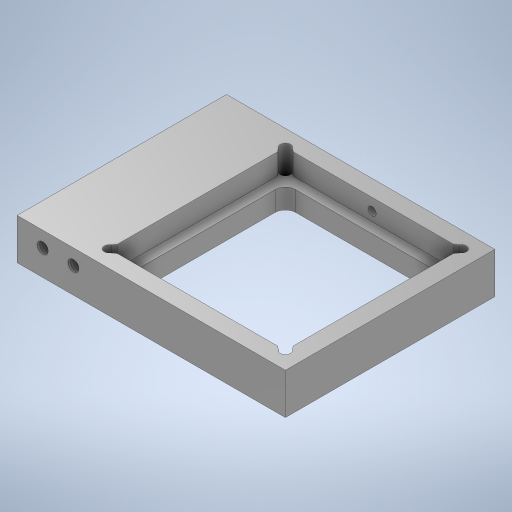
# Autodesk Inventor part: MirrorHolder
Saved by Autodesk Inventor 2023 (Build 270158000, 158)
## iProperties
Created: 2021-10-06
Part Number: MirrorHolder
Material: Aluminum 6061
Document SubType Name: Modeling
Designer: Timo
Density: 2.7 g/cm^3
Appearance: Anodized - Light Gray
Author: Timo
Autodesk Inventor part; units mm, degrees
ref_plane "YZ Plane" through (0, 0, 0) normal (1, 0, 0) x (0, 1, 0)
ref_plane "XZ Plane" through (0, 0, 0) normal (0, 1, 0) x (-1, 0, 0)
ref_plane "XY Plane" through (0, 0, 0) normal (0, 0, 1) x (1, 0, 0)
sketch "Sketch1" plane through (0, 0, 0) normal (0, 1, 0) x (-1, 0, 0)
  line L0 (12, 0) -> (-66.5, 0)
  line L1 (-66.5, 0) -> (-66.5, -61.3)
  line L2 (-66.5, -61.3) -> (12, -61.3)
  line L3 (12, -61.3) -> (12, 0)
  point P0 (0, 0)
  dimension "d0" = 12
  dimension "d1" = 66.5
  dimension "d2" = 61.3
  constraints: 8 end point, 2 parallel, 1 horizontal, 1 perpendicular, 1 point on line
  measures "d0" distance from line of L3 point (0, 0)
  measures "d1" distance from line of L1 point (0, 0)
  measures "d2" distance of L0.end L1.end
extrude "Extrusion1" add sketch "Sketch1" against normal blind 12
sketch "Sketch2" plane through (0, 0, 0) normal (0, 1, 0) x (1, 0, 0)
  line L0 (61.5, 56.5) -> (10, 56.5)
  line L1 (10, 56.5) -> (10, 5)
  line L2 (10, 5) -> (61.5, 5)
  line L3 (61.5, 5) -> (61.5, 56.5)
  line L4 (-12, 0) -> (66.5, 0) projected
  point P0 (0, 0)
  dimension "d5" = 10
  dimension "d6" = 51.5
  dimension "d7" = 5
  dimension "d8" = 51.5
  constraints: 8 end point, 2 parallel, 1 horizontal, 1 perpendicular
  measures "d5" distance from line of point (0, 0) L1
  measures "d6" distance of L2.end L0.start
  measures "d7" distance between parallel lines of L4 L2
  measures "d8" distance of L0.start L0.end
extrude "Extrusion2" cut sketch "Sketch2" against normal blind 6.2
sketch "Sketch3" plane through (0, 0, 0) normal (0, 1, 0) x (1, 0, 0)
  line L0 (61.5, 5) -> (10, 5) projected
  circle A0 centre (10, 5) radius 1.5
  circle A1 centre (61.5, 5) radius 1.5
  line L1 (10, 56.5) -> (61.5, 56.5) projected
  circle A2 centre (61.5, 56.5) radius 1.5
  circle A3 centre (10, 56.5) radius 1.5
  point P0 (0, 0)
  dimension "d11" = 3
  constraints: 4 centre point, 3 equal radius, 2 coincident
  measures "d11" diameter of A0
extrude "Extrusion3" cut sketch "Sketch3" against normal through all
chamfer "Chamfer1" distance 0.8 angle 45 8 edges at (10, -3.1, -6.5) (10, -3.1, -55) (11.5, -3.1, -56.5) (60, -3.1, -56.5) (61.5, -3.1, -55) (61.5, -3.1, -6.5) (60, -3.1, -5) (11.5, -3.1, -5)
sketch "Sketch4" plane through (0, -6.2, 0) normal (0, 1, 0) x (1, 0, 0)
  arc A0 (9.229, 55.2133) -> (11.2867, 57.271) centre (10, 56.5) ccw construction
  line L0 (10, 56.5) -> (61.5, 56.5) construction
  line L1 (61.5, 56.5) -> (61.5, 5) construction
  line L2 (61.5, 5) -> (10, 5) construction
  line L3 (10, 5) -> (10, 56.5) construction
  arc A1 (60.2133, 4.229) -> (62.271, 6.2867) centre (61.5, 5) ccw construction
  line L4 (58.5, 8) -> (58.5, 53.5) construction
  line L5 (58.5, 53.5) -> (13, 53.5) construction
  line L6 (13, 53.5) -> (13, 8) construction
  line L7 (13, 8) -> (58.5, 8) construction
  line L8 (13, 8) -> (58.5, 8)
  line L9 (58.5, 8) -> (58.5, 53.5)
  line L10 (58.5, 53.5) -> (13, 53.5)
  line L11 (13, 53.5) -> (13, 8)
  point P0 (0, 0)
  dimension "d19" = 3
  constraints: 24 end point, 6 parallel, 3 perpendicular, 2 horizontal, 1 coincident, 3 other
  measures "d19" distance between parallel lines of L1 L4
extrude "Extrusion4" cut sketch "Sketch4" against normal blind 6.2
fillet "Fillet1" radius 3 4 edges at (13, -9.1, -53.5) (58.5, -9.1, -8) (13, -9.1, -8) (58.5, -9.1, -53.5)
sketch "Sketch5" plane through (66.5, 0, -61.3) normal (0, 0, -1) x (-1, 0, 0)
  line L0 (0, 0) -> (78.5, 0) projected
  point P0 (66.5, 0)
  point P1 (31.1, -3.5)
  point P2 (56.5, -6.2)
  dimension "d24" = 25.4
  dimension "d25" = 3.5
  measures "d24" horizontal distance of point (56.5, -6.2) point (31.1, -3.5)
  measures "d25" distance from line of L0 point (31.1, -3.5)
hole "Hole1" at (35.4, -3.5, -61.3) direction (0, 0, 1) diameter 2.459 depth 8.8 tip angle 118 thread size "M3x0.5" class "6H" standard "ANSI Metric M Profile"
chamfer "Chamfer2" [suppressed]
sketch "Sketch6" plane through (-12, 0, -61.3) normal (-1, 0, 0) x (0, 0, 1)
  line L0 (56.3, 0) -> (56.3, -6.2) projected
  line L1 (56.3, -6.2) -> (56.3, 0) projected
  line L2 (4.8, -2.2705) -> (4.8, -4.7295) projected
  line L3 (4.8, 0) -> (4.8, -6.2) projected
  line L4 (4.8, -6.2) -> (4.8, 0) projected
  line L5 (30.9, -24.2917) -> (30.9, 19.2353) construction
  line L6 (49.4, 0) -> (12.4, 0) construction
  line L7 (12.4, 0) -> (12.4, -12) construction
  line L8 (12.4, -12) -> (49.4, -12) construction
  line L9 (49.4, -12) -> (49.4, 0) construction
  line L10 (49.4, 0) -> (12.4, -12) construction
  line L11 (12.4, 0) -> (49.4, -12) construction
  line L12 (0, 0) -> (61.3, 0) projected
  line L13 (61.3, -12) -> (0, -12) projected
  line L14 (7.1, -6.2) -> (54, -6.2) projected
  point P0 (30.9, -6)
  point P1 (19.7, -6.2)
  point P2 (42.1, -6.2)
  dimension "d36" = 25.4
  dimension "d37" = 37
  dimension "d38" = 22.4
  constraints: 14 end point, 5 point on line, 2 midpoint, 2 parallel, 1 horizontal, 1 perpendicular, 1 symmetric about line, 1 vertical
  measures "d36" distance between parallel lines of L0 L5
  measures "d37" distance of L7.end L8.end
  measures "d38" distance of point (19.7, -6.2) point (42.1, -6.2)
hole "Hole2" at (-12, -6.2, -41.6) at (-12, -6.2, -19.2) at (-12, -6, -30.4) direction (1, 0, 0) diameter 3.242 depth 11.8 tip angle 118 thread size "M4x0.7" class "6H" standard "ANSI Metric M Profile"
sketch "Sketch7" plane through (-12, 0, 0) normal (0, 0, 1) x (1, 0, 0)
  line L0 (0, 0) -> (78.5, 0) projected
  line L1 (16.5, -4.5) -> (7.5, -4.5) construction
  point P0 (12, 0)
  dimension "d52" = 9
  dimension "d53" = 4.5
  dimension "d54" = 4.5
  constraints: 2 end point, 1 horizontal
  measures "d52" distance of L1.end L1.start
  measures "d53" distance from line of L0 L1.start
  measures "d54" horizontal distance of L1.end point (12, 0)
hole "Hole3" at (-4.5, -4.5, 0) at (4.5, -4.5, 0) direction (0, 0, -1) diameter 3.242 depth 11.8 tip angle 118 thread size "M4x0.7" class "6H" standard "ANSI Metric M Profile"
equation "\"d54\" = 0.5 * d52"
body "Solid1"
